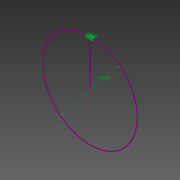
# Autodesk Inventor part: Sketch curvatura
Saved by Autodesk Inventor 2019 (Build 230136000, 136)
## iProperties
Created: 2019-10-31
Part Number: Sketch curvatura
Material: Generic
Document SubType Name: Modeling
Designer: Charlie
Density: 1 g/cm^3
Appearance: Default
Author: Charlie
Autodesk Inventor part; units mm, degrees
ref_plane "YZ Plane" through (0, 0, 0) normal (1, 0, 0) x (0, 1, 0)
ref_plane "XZ Plane" through (0, 0, 0) normal (0, 1, 0) x (-1, 0, 0)
ref_plane "XY Plane" through (0, 0, 0) normal (0, 0, 1) x (1, 0, 0)
sketch "Sketch1" plane through (0, 0, 0) normal (0, 0, 1) x (1, 0, 0)
  line L0 (-327.5, 21447.5) -> (327.5, 21447.5)
  line L1 (327.5, 21447.5) -> (327.5, 21287.5)
  line L2 (327.5, 21287.5) -> (-327.5, 21287.5)
  line L3 (-327.5, 21287.5) -> (-327.5, 21447.5)
  circle A0 centre (0, 0) radius 21452.5
  line L4 (-327.5, 21447.5) -> (-327.5, 21450)
  line L5 (327.5, 21447.5) -> (327.5, 21450)
  circle A1 centre (0, 0) radius 21552.5
  circle A2 centre (0, 0) radius 21592.5
  line L6 (0, 0) -> (-390.0286, 21448.9541)
  line L7 (0, 0) -> (390.0286, 21448.9541)
  circle A3 centre (-331.1139, 21519.9528) radius 30
  circle A4 centre (-286.1898, 21600.6042) radius 10
  circle A5 centre (-378.498, 21599.1839) radius 10
  line L8 (-378.498, 21599.1839) -> (-331.1139, 21519.9528) construction
  line L9 (-331.1139, 21519.9528) -> (-286.1898, 21600.6042) construction
  line L10 (-378.498, 21599.1839) -> (-286.1898, 21600.6042) construction
  line L11 (-331.1139, 21519.9528) -> (-330.037, 21449.9611) construction
  line L12 (-391.8781, 21548.937) -> (-392.6178, 21588.9302)
  line L13 (-390.0286, 21448.9541) -> (-391.8781, 21548.937) construction
  line L14 (390.0286, 21448.9541) -> (391.8781, 21548.937) construction
  line L15 (391.8781, 21548.937) -> (392.6178, 21588.9302)
  ellipse E0 centre (0, 21447.5) end of major axis (327.5, 21447.5) minor radius 5
  dimension "d0" = 655
  dimension "d1" = 160
  dimension "d2" = 42905
  dimension "d3" = 2.5
  dimension "d4" = 40
  dimension "d5" = 100
  dimension "d7" = 1.042
  dimension "d8" = 20
  dimension "d9" = 60
  dimension "d13" = 60
  dimension "d14" = 1.042
  constraints: 32 end point, 9 point on circle, 6 centre point, 3 coincident, 3 equal length, 3 tangent, 2 collinear, 2 horizontal, 2 parallel, 2 vertical, 1 equal radius, 1 horizontal alignment, 1 line through centre, 1 midpoint, 1 perpendicular, 2 other
  measures "d0" distance of L1.end L2.end
  measures "d1" distance of L0.end L1.end
  measures "d2" diameter of A0
  measures "d3" distance of L0.start L4.end
  measures "d4" radial gap between concentric circles of A1 A2
  measures "d5" radial gap between concentric circles of A0 A1
  measures "d7" angle of L1 L7
  measures "d8" diameter of A4
  measures "d9" diameter of A3
  measures "d13" distance from line of L13 L11.end
  measures "d14" angle of L6 L3
extrude "Extrusion1" add sketch "Sketch1" along normal blind 20 contours A1 L12 A2 L15 picked at (-256.116, 21564.1758)
equation "\"d7\" = d14"
body "Solid1"
